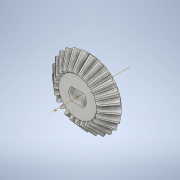
# Autodesk Inventor part: Wechsel_Kegelrad2
Saved by Autodesk Inventor 2021 (Build 250183000, 183)
## iProperties
CustomPartVersion: 1
Created: 2021-01-24
Part Number: Wechsel_Kegelrad2
Material: Steel, Mild
Document SubType Name: Modeling
Designer: Jaro Machnow
Categories: <?xml version="1.0" encoding="UTF-16"?> <MemberInstance><Categories><FamilyTemplate><FamilyTemplateParameter ValueType="xs:double" Id="1" ObjectReferenceKey="da_z" ObjectType="kUserParameterObject"/><FamilyTemplateParameter ValueType="xs:double" Id="2" ObjectReferenceKey="da_b" ObjectType="kUserParameterObject"/><FamilyTemplateParameter ValueType="xs:double" Id="3" ObjectReferenceKey="da_beta" ObjectType="kUserParameterObject"/><FamilyTemplateParameter ValueType="xs:double" Id="4" ObjectReferenceKey="da_dae" ObjectType="kUserParameterObject"/><FamilyTemplateParameter ValueType="xs:double" Id="5" ObjectReferenceKey="da_ve" ObjectType="kUserParameterObject"/><FamilyTemplateParameter ValueType="xs:double" Id="6" ObjectReferenceKey="da_omega" ObjectType="kUserParameterObject"/><FamilyTemplateParameter ValueType="xs:string" Id="7" ObjectReferenceKey="EAIAABAAAAAAHwAAAAAAAIAAAAAAAAAA" ObjectType="83914240" SubObjectId="SurfaceGeometry"/></FamilyTemplate><ParamToTemplateMap><ParamToTemplate CategoryParameter="//CategoryParameter[@InternalName='046C89C9-8512-4d59-83FE-43B91F4F132A']" TemplateParameter="1"/><ParamToTemplate CategoryParameter="//CategoryParameter[@InternalName='2552DF32-E462-4b46-AEBF-C6C7768E72AC']" TemplateParameter="2"/><ParamToTemplate CategoryParameter="//CategoryParameter[@InternalName='C9EE641D-15FC-4fae-A226-E94C4372FDD7']" TemplateParameter="3"/><ParamToTemplate><ParamToTemplate CategoryParameter="//CategoryParameter[@InternalName='00B6519A-459B-49c7-AD84-2E56D39A5744']" ConstantValue="-0.000000"/></ParamToTemplate><ParamToTemplate><ParamToTemplate CategoryParameter="//CategoryParameter[@InternalName='04B31F0E-C7A6-4894-AA32-9629BEFACF47']" ConstantValue="1.000000"/></ParamToTemplate><ParamToTemplate><ParamToTemplate CategoryParameter="//CategoryParameter[@InternalName='43CBEC2E-7847-49e7-A936-2F7889FCB2D9']" ConstantValue="0.200000"/></ParamToTemplate><ParamToTemplate><ParamToTemplate CategoryParameter="//CategoryParameter[@InternalName='B1EFC894-105D-4ebd-86BF-FA20ED196853']" ConstantValue="0.300000"/></ParamToTemplate><ParamToTemplate><ParamToTemplate CategoryParameter="//CategoryParameter[@InternalName='51175063-3D10-4879-93E8-6246FE8B403D']" ConstantValue="2060000000.000000"/></ParamToTemplate><ParamToTemplate><ParamToTemplate CategoryParameter="//CategoryParameter[@InternalName='A3A52E27-4454-46a9-B0BD-C932399B70AF']" ConstantValue="0.300000"/></ParamToTemplate><ParamToTemplate CategoryParameter="//CategoryParameter[@InternalName='2A200944-5A8C-41ca-B96E-8520D2E510F1']" TemplateParameter="4"/><ParamToTemplate><ParamToTemplate CategoryParameter="//CategoryParameter[@InternalName='1A637F62-92C8-44bc-B81F-10802510B579']" ConstantValue="2.467918"/></ParamToTemplate><ParamToTemplate CategoryParameter="//CategoryParameter[@InternalName='B52DD4BE-6863-48fb-BF58-89EF6F9EC65C']" TemplateParameter="5"/><ParamToTemplate><ParamToTemplate CategoryParameter="//CategoryParameter[@InternalName='3956BFF2-84D2-457d-93C2-9B0613DEBA67']" ConstantValue="1.101827"/></ParamToTemplate><ParamToTemplate CategoryParameter="//CategoryParameter[@InternalName='739CFA02-461B-4bf8-8049-181FCAD8B28F']" TemplateParameter="6"/><ParamToTemplate><ParamToTemplate CategoryParameter="//CategoryParameter[@InternalName='A27E999F-E2CE-4481-8A2A-EBF499C4C3C5']" ConstantValue="-0.000000"/></ParamToTemplate><ParamToTemplate><ParamToTemplate CategoryParameter="//CategoryParameter[@InternalName='9E1B4470-B2D3-4ff1-B813-535BB4CDF51A']" ConstantValue="3520000.000000"/></ParamToTemplate><ParamToTemplate><ParamToTemplate CategoryParameter="//CategoryParameter[@InternalName='F8452263-BFF6-458c-9FB1-07C4B99E95CD']" ConstantValue="11400000.000000"/></ParamToTemplate><ParamToTemplate><ParamToTemplate CategoryParameter="//CategoryParameter[@InternalName='3E3BB259-FD49-497f-8171-6EBC954A3479']" ConstantValue="2.000000"/></ParamToTemplate><ParamToTemplate CategoryParameter="//CategoryParameter[@InternalName='27C3BAF2-7550-4e4b-AE2C-0DB134B7D9B7']" TemplateParameter="7"/></ParamToTemplateMap><Category DisplayName="Gear" InternalName="DC85795E-93AB-48d5-8EEE-5A27447B64BD" Mnemonic="Gear"><CategoryParameter DisplayName="z" InternalName="046C89C9-8512-4d59-83FE-43B91F4F132A" Mnemonic="z"/><CategoryParameter DisplayName="b" InternalName="2552DF32-E462-4b46-AEBF-C6C7768E72AC" Mnemonic="b"/><CategoryParameter DisplayName="||b|" InternalName="C9EE641D-15FC-4fae-A226-E94C4372FDD7" Mnemonic="beta"/><CategoryParameter DisplayName="x" InternalName="00B6519A-459B-49c7-AD84-2E56D39A5744" Mnemonic="x"/><CategoryParameter DisplayName="a*" InternalName="04B31F0E-C7A6-4894-AA32-9629BEFACF47" Mnemonic="a"/><CategoryParameter DisplayName="c*" InternalName="43CBEC2E-7847-49e7-A936-2F7889FCB2D9" Mnemonic="c"/><CategoryParameter DisplayName="r|.f|*" InternalName="B1EFC894-105D-4ebd-86BF-FA20ED196853" Mnemonic="rf"/><CategoryParameter DisplayName="E" InternalName="51175063-3D10-4879-93E8-6246FE8B403D" Mnemonic="E"/><CategoryParameter DisplayName="||m|" InternalName="A3A52E27-4454-46a9-B0BD-C932399B70AF" Mnemonic="mi"/><Category DisplayName="BevelGear" InternalName="0C98F69A-0C2B-4791-B2FE-7691BB227E77" Mnemonic="BevelGear"><CategoryParameter DisplayName="d|.ae|" InternalName="2A200944-5A8C-41ca-B96E-8520D2E510F1" Mnemonic="dae"/><CategoryParameter DisplayName="d|.ai|" InternalName="1A637F62-92C8-44bc-B81F-10802510B579" Mnemonic="dai"/><CategoryParameter DisplayName="A|.e|" InternalName="B52DD4BE-6863-48fb-BF58-89EF6F9EC65C" Mnemonic="ve"/><CategoryParameter DisplayName="A|.i|" InternalName="3956BFF2-84D2-457d-93C2-9B0613DEBA67" Mnemonic="vi"/><CategoryParameter DisplayName="||S|" InternalName="739CFA02-461B-4bf8-8049-181FCAD8B28F" Mnemonic="omega"/><CategoryParameter DisplayName="x|.t|" InternalName="A27E999F-E2CE-4481-8A2A-EBF499C4C3C5" Mnemonic="xt"/><CategoryParameter DisplayName="||s||.Flim|" InternalName="9E1B4470-B2D3-4ff1-B813-535BB4CDF51A" Mnemonic="sFlim"/><CategoryParameter DisplayName="||s||.Hlim|" InternalName="F8452263-BFF6-458c-9FB1-07C4B99E95CD" Mnemonic="sHlim"/><CategoryParameter DisplayName="Typ" InternalName="3E3BB259-FD49-497f-8171-6EBC954A3479" Mnemonic="type"/><CategoryParameter DisplayName="PitchDiameter" InternalName="27C3BAF2-7550-4e4b-AE2C-0DB134B7D9B7" Mnemonic="IDS_PITCHDIAM"/></Category></Category></Categories></MemberInstance>
Mass: 60.9118 g
Surface Area: 34.3074 cm^2
Volume: 7.7496 cm^3
Density: 7.86 g/cm^3
Appearance: Steel
Author: Jaro Machnow
Autodesk Inventor part; units mm, degrees
ref_plane "Netzebene2" through (0, 0, 0) normal (0.9921147, 0.1253332, 0) x (0, 0, 1)
sketch "Skizze des Zahnradkörpers" plane through (0, 0, 0) normal (1, 0, 0) x (0, 1, 0)
  line L0 (0, 0) -> (17.477208, -20.022792) construction
  line L1 (17.477208, -20.022792) -> (19.81066, -17.68934)
  line L2 (19.81066, -17.68934) -> (0, 0) construction
  line L3 (18.75, -18.75) -> (0, 0) construction
  line L4 (10.88614, -12.471724) -> (12.339592, -11.018272)
  line L5 (17.477208, -20.022792) -> (10.88614, -12.471724)
  line L6 (19.81066, -17.68934) -> (12.339592, -11.018272)
  line L7 (0, -37.144798) -> (0, 6.1908)
  line L8 (0, -18.75) -> (19.81066, -18.75) construction
  dimension "d0" = 37.5
  dimension "d1" = 34.95442
  dimension "d2" = 39.62132
  dimension "d3" = 10
  dimension "d4" = 17.68934
  constraints: 16 end point, 4 point on line, 3 perpendicular, 2 collinear, 1 horizontal alignment, 1 vertical alignment
  measures "d0" diameter of L3.start L7
  measures "d1" diameter of L0.end L7
  measures "d2" diameter of L1.end L7
  measures "d3" distance between parallel lines of L1 L4
  measures "d4" vertical distance of L1.end L0.start
revolve "Zahnradkörper" add sketch "Skizze des Zahnradkörpers" angle 360 about axis through (0, 0, 0) along (0, 0, 1)
ref_plane "Zahnebene" through (0, 18.75, -18.75) normal (0, -0.7071068, 0.7071068) x (1, 0, 0)
sketch "Startskizze" plane through (0, 18.75, -18.75) normal (0, -0.7071068, 0.7071068) x (1, 0, 0)
  line L0 (0, -27.034511) -> (0, 7.43081)
  arc A0 (-0.574804, -2.196) -> (-2.631161, 2.370418) centre (-10.037026, -3.710823) ccw
  arc A1 (2.631161, 2.370418) -> (0.574804, -2.196) centre (10.037026, -3.710823) ccw
  line L1 (-0.574804, -2.196) -> (0.574804, -2.196)
  arc A2 (2.631161, 2.370418) -> (-2.631161, 2.370418) centre (0, -26.516504) ccw
  dimension "d7" = 9.58271
  dimension "d8" = 10.03703
  dimension "d9" = 22.80568
  dimension "d57" = 29.0065
  dimension "d58" = 24.3205
  constraints: 6 point on circle, 3 centre point, 3 symmetric about line, 2 end point, 1 coincident, 1 perpendicular, 1 other
  measures "d7" radius of A0
  measures "d8" horizontal distance of point (0, -26.517) A0.centre
  measures "d9" vertical distance of point (0, -26.517) A0.centre
  measures "d57" radius of A2
  measures "d58" distance from line of A2.centre L1
ref_plane "Endebene" through (0, 11.56226, -11.56226) normal (0, -0.7071068, 0.7071068) x (1, 0, 0)
sketch "Endskizze" plane through (0, 11.56226, -11.56226) normal (0, -0.7071068, 0.7071068) x (1, 0, 0)
  line L0 (0, -19.266682) -> (0, 5.295715)
  arc A0 (-0.354455, -1.354172) -> (-1.622515, 1.461727) centre (-6.189371, -2.288294) ccw
  arc A1 (1.622515, 1.461727) -> (0.354455, -1.354172) centre (6.189371, -2.288294) ccw
  line L1 (-0.354455, -1.354172) -> (0.354455, -1.354172)
  arc A2 (1.622515, 1.461727) -> (-1.622515, 1.461727) centre (0, -16.351504) ccw
  dimension "d12" = 5.90922
  dimension "d15" = 6.18937
  dimension "d16" = 14.06321
  dimension "d59" = 17.88697
  dimension "d60" = 14.99733
  constraints: 6 point on circle, 3 centre point, 3 symmetric about line, 2 end point, 1 coincident, 1 other
  measures "d12" radius of A0
  measures "d15" horizontal distance of A0.centre point (0, -16.352)
  measures "d16" vertical distance of A0.centre point (0, -16.352)
  measures "d59" radius of A2
  measures "d60" distance from line of A2.centre L1
loft "Loft" cut profiles "Startskizze", "Endskizze"
pattern_circular "Circular Pattern" count 25 over 360 about axis through (0, 0, 0) along (0, 0, 1) of "Loft"
sketch3d "3D-Skizze rechts"
ref_plane "Endebene rechts" through (-3.895095, 10.886417, -11.56226) normal (0.2382102, -0.6657747, 0.7071068) x (0.9415476, 0.3368801, 0)
sketch "Endskizze rechts" plane through (-3.895095, 10.886417, -11.56226) normal (0.2382102, -0.6657747, 0.7071068) x (0.9415476, 0.3368801, 0)
  arc A0 (-0.354455, -1.354172) -> (-1.622515, 1.461727) centre (-6.189371, -2.288294) ccw
  line L0 (0, -23.830182) -> (0, 9.265479)
  arc A1 (1.622515, 1.461727) -> (0.354455, -1.354172) centre (6.189371, -2.288294) ccw
  line L1 (-0.354455, -1.354172) -> (0.354455, -1.354172)
  arc A2 (1.622515, 1.461727) -> (-1.622515, 1.461727) centre (0, -16.351504) ccw
  dimension "d70" = 6.18937
  dimension "d71" = 14.06321
  dimension "d72" = 5.90922
  dimension "d73" = 14.99733
  dimension "d74" = 17.88697
  constraints: 6 point on circle, 3 centre point, 3 symmetric about line, 2 end point, 1 coincident, 1 perpendicular, 1 other
  measures "d70" horizontal distance of A2.centre A0.centre
  measures "d71" vertical distance of point (0, -16.352) A0.centre
  measures "d72" radius of A0
  measures "d73" distance from line of point (0, -16.352) L1
  measures "d74" radius of A2
feature "Erhebung rechts" [suppressed]
pattern_circular "Runde Anordnung rechts" [suppressed]
sketch3d "3D-Skizze links"
ref_plane "Endebene links" through (3.748133, 10.886417, -11.484542) normal (-0.2304821, -0.6694331, 0.7062133) x (0.9455282, -0.3255401, 0)
sketch "Endskizze links" plane through (3.748133, 10.886417, -11.484542) normal (-0.2304821, -0.6694331, 0.7062133) x (0.9455282, -0.3255401, 0)
  line L0 (0, -37.037572) -> (0, 15.545753)
  arc A0 (-0.354455, -1.374806) -> (-1.622515, 1.441093) centre (-6.189371, -2.308928) ccw
  arc A1 (1.622515, 1.441093) -> (0.354455, -1.374806) centre (6.189371, -2.308928) ccw
  line L1 (-0.354455, -1.374806) -> (0.354455, -1.374806)
  ellipse E0 centre (0, -7.800927) end of major axis (12.339592, -7.800927) minor radius 8.714385
  arc A2 (1.622515, 1.441093) -> (-1.622515, 1.441093) centre (0, -16.372139) ccw
  dimension "d56" = 8.71438
  dimension "d30" = 5.90922
  dimension "d31" = 6.18937
  dimension "d32" = 14.06321
  dimension "d61" = 17.88697
  dimension "d62" = 14.99733
  constraints: 6 point on circle, 3 centre point, 3 symmetric about line, 2 end point, 1 coincident, 2 other
  measures "d30" radius of A0
  measures "d31" horizontal distance of point (0, -16.372) A0.centre
  measures "d32" vertical distance of A0.centre point (0, -16.372)
  measures "d61" radius of A2
  measures "d62" distance from line of point (0, -16.372) L1
feature "Erhebung links" [suppressed]
pattern_circular "Runde Anordnung links" [suppressed]
sketch "Körperskizze" plane through (0, 0, 0) normal (1, 0, 0) x (0, 1, 0)
  line L0 (0, -32.703927) -> (0, -20.454423)
  line L1 (17.477208, -20.022792) -> (10.88614, -12.471724)
  line L2 (10.88614, -12.471724) -> (0, -12.471724)
  line L3 (17.477208, -20.022792) -> (0, -20.022792)
  constraints: 4 end point, 2 perpendicular, 2 point on line
sketch "Körperskizze outline for Festkörper" plane through (0, 0, 0) normal (1, 0, 0) x (0, 1, 0)
  line L0 (0, -20.022792) -> (17.477208, -20.022792)
  line L1 (0, -12.471724) -> (0, -20.022792)
  line L2 (10.88614, -12.471724) -> (0, -12.471724)
  line L3 (17.477208, -20.022792) -> (10.88614, -12.471724)
revolve "Festkörper" add sketch "Körperskizze outline for Festkörper" angle 360 about axis through (0, 0, 0) along (0, 0, 1)
sketch "Sketch6" plane through (0, 0, 0) normal (1, 0, 0) x (0, 1, 0)
  line L0 (18.75, -18.75) -> (0, 0) projected
  line L1 (0, -36) -> (0, 6) projected
surface revolve "Flankendurchmesser" sketch "Sketch6" angle 360 about axis through (0, 0, 0) along (0, 0, 1) shown no curves L0
sketch "Skizze8" plane through (0, 0, -12.471724) normal (0, 0, 1) x (1, 0, 0)
  line L0 (-3.570714, 3.5) -> (3.570714, 3.5)
  line L1 (3.570714, 3.5) -> (-3.570714, 3.5)
  line L2 (3.570714, -3.5) -> (-3.570714, -3.5)
  arc A0 (-3.570714, 3.5) -> (-3.570714, -3.5) centre (0, 0) ccw
  arc A1 (3.570714, -3.5) -> (3.570714, 3.5) centre (0, 0) ccw
  constraints: 6 end point, 4 point on circle, 2 centre point, 1 coincident, 1 collinear, 1 horizontal
extrude "Extrusion1" cut sketch "Skizze8" against normal blind 10
equation "\"d0\" = da_de"
equation "\"d1\" = da_dfe"
equation "\"d2\" = da_dae"
equation "\"d3\" = da_b"
equation "\"d4\" = da_ve"
equation "\"d7\" = fd_rr"
equation "\"d8\" = fd_x"
equation "\"d9\" = fd_y"
equation "\"d57\" = 0.5 * fd_dva + 0.3 * da_he"
equation "\"d58\" = 0.5 * fd_dva - 1.12 * da_he"
equation "\"da_teethtype\" = 0"
equation "\"da_b\" = 10"
equation "\"da_de\" = 37.5"
equation "\"da_dae\" = 39.62132"
equation "\"da_dfe\" = 34.95442"
equation "\"da_le\" = 26.5165"
equation "\"da_omega\" = 90deg"
equation "\"da_beta\" = 0"
equation "\"da_delta\" = 45deg"
equation "\"da_alpha\" = 20deg"
equation "\"da_he\" = 3.3"
equation "\"da_ve\" = 17.68934"
equation "\"da_zv\" = 35.355339"
equation "\"fd_loft\" = da_b + 0.05 * da_he"
equation "\"fd_x\" = fd_x1 + fd_x2"
equation "\"fd_y\" = fd_y1 - fd_y2"
equation "\"fd_dd\" = fd_dva - 0.8 * da_he"
equation "\"da_dvw\" = 53.03301"
equation "\"d11\" = fd_loft"
equation "\"da_dm\" = 30.42893"
equation "\"da_x\" = 0"
equation "\"da_m\" = 1.5"
equation "\"d50\" = da_omega"
equation "\"fd_rr\" = 9.582711"
equation "\"fd_dva\" = 56.033009"
equation "\"fd_x1\" = 1.190787"
equation "\"fd_x2\" = 8.846239"
equation "\"fd_y1\" = 26.489753"
equation "\"fd_y2\" = 3.684072"
body "Solid1"
body "Srf1"
